Spring for bed leveling (Autodesk Fusion 360 design; units mm, degrees)
Autodesk Fusion 360 part; units mm, degrees
coil "CoilPrimitive1" add diameter 4 section square size 1 outside turns 10 pitch 2 right hand placed x (1, 0, 0) y (0, 1, 0) z (0, 0, 1) at (0, 0, 0)
